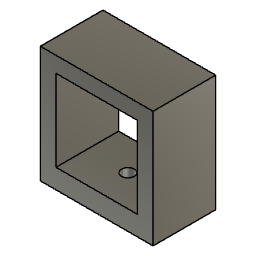
Arm Base Attachment v4 (Autodesk Fusion 360 design; units mm, degrees)
Autodesk Fusion 360 part; units mm, degrees
sketch "Sketch1" plane through (0, 0, 0) normal (0, 0, 1) x (1, 0, 0)
  line L0 (18.288, -10.16) -> (-18.288, -10.16)
  line L1 (-18.288, -10.16) -> (-18.288, 10.16)
  line L2 (-18.288, 10.16) -> (18.288, 10.16)
  line L3 (18.288, 10.16) -> (18.288, -10.16)
  line L4 (18.288, -10.16) -> (-18.288, 10.16) construction
  line L5 (-18.288, -10.16) -> (18.288, 10.16) construction
  circle A0 centre (0, 0) radius 2.0574
  dimension "d1" = 36.576
  dimension "d2" = 20.32
  dimension "d3" = 4.1148
  constraint horizontal L0
  constraint perpendicular L0 L1
  constraint parallel L0 L2
  constraint parallel L1 L3
  constraint coincident L4 A0.centre
  constraint coincident L5 A0.centre
  constraint coincident A0.centre origin
  measures "d1" distance of L1.end L2.end
  measures "d2" distance of L0.start L2.end
  measures "d3" diameter of A0
extrude "Extrude1" add sketch "Sketch1" along normal blind 6.35
sketch "Sketch2" plane through (0, 0, 6.35) normal (0, 0, 1) x (-1, 0, 0)
  circle A0 centre (0, 0) radius 2.0574
  line L0 (-18.288, -10.16) -> (18.288, -10.16)
  line L1 (18.288, -10.16) -> (18.288, 10.16)
  line L2 (18.288, 10.16) -> (-18.288, 10.16)
  line L3 (-18.288, 10.16) -> (-18.288, -10.16)
  line L4 (18.288, -10.16) -> (13.208, -10.16)
  line L5 (13.208, -10.16) -> (13.208, 10.16)
  line L6 (13.208, 10.16) -> (18.288, 10.16)
  line L7 (18.288, -10.16) -> (18.288, 10.16)
  line L8 (-18.288, -10.16) -> (-13.208, -10.16)
  line L9 (-13.208, -10.16) -> (-13.208, 10.16)
  line L10 (-13.208, 10.16) -> (-18.288, 10.16)
  line L11 (-18.288, -10.16) -> (-18.288, 10.16)
  dimension "d6" = 5.08
  dimension "d7" = 5.08
  constraint coincident L0.end L1.start
  constraint perpendicular L1 L4
  constraint coincident L2 L5.end
  constraint perpendicular L2 L5
  constraint coincident L1.end L2.start
  constraint coincident L0.start L3.end
  constraint perpendicular L5 L8
  constraint coincident L2 L9.end
  constraint perpendicular L2 L9
  constraint coincident L2.end L3.start
  measures "d6" distance of L0.end L4.end
  measures "d7" distance of L0.start L8.end
extrude "Extrude2" add sketch "Sketch2" along normal blind 26.416 contours L0 L2 L3 L8 L9 L10 L11 | L0 L1 L2 L4 L5 L6 L7
sketch "Sketch3" plane through (0, 0, 32.766) normal (0, 0, 1) x (-1, 0, 0)
  line L0 (13.208, -10.16) -> (18.288, -10.16)
  line L1 (18.288, -10.16) -> (18.288, 10.16)
  line L2 (18.288, 10.16) -> (13.208, 10.16)
  line L3 (13.208, 10.16) -> (13.208, -10.16)
  line L4 (18.288, -10.16) -> (-18.288, -10.16)
  line L5 (-18.288, -10.16) -> (-18.288, 10.16)
  line L6 (-18.288, 10.16) -> (18.288, 10.16)
  line L7 (18.288, 10.16) -> (18.288, -10.16)
  point P0 (-18.288, 10.16)
  dimension "d10" = 20.32
  dimension "d11" = 36.576
  constraint horizontal L4
  constraint vertical L5
  constraint horizontal L6
  constraint vertical L7
  constraint coincident L0.end L1.start
  constraint coincident P0 L5.end
  measures "d10" distance of L4.end P0
  measures "d11" distance of P0 L1.end
extrude "Extrude3" add sketch "Sketch3" along normal blind 5.08
